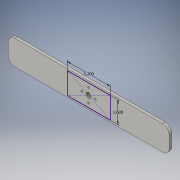
# Autodesk Inventor part: New_Top
Saved by Autodesk Inventor 2016 (Build 200138000, 138)
## iProperties
Created: 2018-05-03
Part Number: New_Top
Material: Generic
Document SubType Name: Modeling
Designer: student
Density: 1 g/cm^3
Appearance: Default
Author: student
Autodesk Inventor part; units mm, degrees
ref_plane "YZ Plane" through (0, 0, 0) normal (1, 0, 0) x (0, 1, 0)
ref_plane "XZ Plane" through (0, 0, 0) normal (0, 1, 0) x (-1, 0, 0)
ref_plane "XY Plane" through (0, 0, 0) normal (0, 0, 1) x (1, 0, 0)
sketch "Sketch1" plane through (0, 0, 0) normal (0, 0, 1) x (1, 0, 0)
  line L0 (-152.4, -23.495) -> (152.4, -23.495)
  line L1 (152.4, -23.495) -> (152.4, 23.495)
  line L2 (152.4, 23.495) -> (-152.4, 23.495)
  line L3 (-152.4, 23.495) -> (-152.4, -23.495)
  line L4 (-152.4, -23.495) -> (152.4, 23.495) construction
  line L5 (152.4, -23.495) -> (-152.4, 23.495) construction
  point P0 (0, 0)
  dimension "d0" = 304.8
  dimension "d1" = 46.99
  constraints: 12 end point, 2 midpoint, 2 parallel, 1 horizontal, 1 perpendicular
  measures "d0" distance of L2.end L1.end
  measures "d1" distance of L1.end L0.end
extrude "Extrusion1" add sketch "Sketch1" along normal blind 5.08
fillet "Fillet1" radius 12.7 4 edges at (152.4, 23.495, 2.54) (152.4, -23.495, 2.54) (-152.4, 23.495, 2.54) (-152.4, -23.495, 2.54)
sketch "Sketch2" plane through (0, 0, 5.08) normal (0, 0, 1) x (1, 0, 0)
  line L0 (-40.64, -20.32) -> (40.64, -20.32)
  line L1 (40.64, -20.32) -> (40.64, 20.32)
  line L2 (40.64, 20.32) -> (-40.64, 20.32)
  line L3 (-40.64, 20.32) -> (-40.64, -20.32)
  line L4 (-40.64, -20.32) -> (40.64, 20.32) construction
  line L5 (40.64, -20.32) -> (-40.64, 20.32) construction
  point P0 (0, 0)
  dimension "d5" = 81.28
  dimension "d6" = 40.64
  constraints: 12 end point, 2 midpoint, 2 parallel, 1 horizontal, 1 perpendicular
  measures "d5" distance of L2.end L1.end
  measures "d6" distance of L1.end L0.end
sketch "Sketch3" plane through (0, 0, 5.08) normal (0, 0, 1) x (1, 0, 0)
  circle A0 centre (0, 12.7) radius 1.6891
  circle A1 centre (0, -12.7) radius 1.6891
  circle A2 centre (12.7, 0) radius 1.6891
  circle A3 centre (-12.7, 0) radius 1.6891
  circle A4 centre (0, 0) radius 4.699
  point P0 (0, 0)
  point P1 (0, 0)
  dimension "d7" = 3.3782
  dimension "d8" = 3.3782
  dimension "d9" = 3.3782
  dimension "d10" = 3.3782
  dimension "d11" = 9.398
  dimension "d12" = 12.7
  dimension "d13" = 12.7
  dimension "d14" = 12.7
  dimension "d15" = 12.7
  dimension "d16" = 0
  constraints: 5 centre point
  measures "d7" diameter of A0
  measures "d8" diameter of A1
  measures "d9" diameter of A2
  measures "d10" diameter of A3
  measures "d11" diameter of A4
  measures "d12" distance of point (0, 0) A0.centre
  measures "d13" distance of point (0, 0) A2.centre
  measures "d14" distance of A4.centre A1.centre
  measures "d15" distance of A3.centre point (0, 0)
  measures "d16" distance of point (0, 0) A4.centre
extrude "Extrusion2" cut sketch "Sketch3" against normal blind 5.08
body "Solid1"
